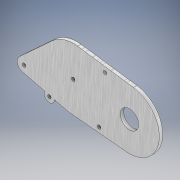
# Autodesk Inventor part: 後脚ギアトレイン5.1
Saved by Autodesk Inventor 2020 (Build 240168000, 168)
## iProperties
Created: 2019-09-03
Part Number: 後脚ギアトレイン5.1
Material: アルミニウム 7075
Document SubType Name: Modeling
Designer: 雪村
Density: 2.81 g/cm^3
Appearance: サテン - ブラシ仕上げ 重厚
Mass: 43.3309 g
Surface Area: 115.743 cm^2
Volume: 15.4203 cm^3
Author: 雪村
Autodesk Inventor part; units mm, degrees
ref_plane "YZ Plane" through (0, 0, 0) normal (1, 0, 0) x (0, 1, 0)
ref_plane "XZ Plane" through (0, 0, 0) normal (0, 1, 0) x (-1, 0, 0)
ref_plane "XY Plane" through (0, 0, 0) normal (0, 0, 1) x (1, 0, 0)
sketch "スケッチ1" plane through (0, 0, 0) normal (0, 0, 1) x (1, 0, 0)
  circle A0 centre (-27.1196, 80) radius 1.5
  circle A1 centre (-27.1196, 80) radius 6
  circle A2 centre (20.6799, 65) radius 1.5
  circle A3 centre (20.6799, 65) radius 6
  circle A4 centre (63.5417, 75.7941) radius 1.5
  circle A5 centre (-68.1796, 83.3936) radius 1.5
  circle A6 centre (-112.5, 70) radius 8.025
  circle A7 centre (112.5, 70) radius 8.025
  arc A8 (109.9686, 44.1235) -> (116.0788, 95.7525) centre (112.5, 70) ccw
  circle A9 centre (-94.9808, 96.6696) radius 4.5
  circle A10 centre (-94.9808, 96.6696) radius 1.5
  circle A11 centre (-83.1426, 57.4965) radius 1.5
  circle A12 centre (-83.1426, 57.4965) radius 4.5
  circle A13 centre (86.1018, 50.9798) radius 4.5
  circle A14 centre (86.1018, 50.9798) radius 1.5
  circle A15 centre (91.2708, 94.6568) radius 1.5
  circle A16 centre (91.2708, 94.6568) radius 4.5
  line L0 (-103.9107, 45.4598) -> (-60.251, 60.7411)
  line L1 (-118.9391, 95.19) -> (-74.1234, 106.646)
  line L2 (-55.9515, 104.0449) -> (-24.0626, 85.1628)
  line L3 (-24.9517, 74.4053) -> (-59.508, 61.015)
  line L4 (116.0788, 95.7525) -> (67.2581, 102.5371)
  line L5 (45.3001, 95.7) -> (16.6263, 69.4235)
  line L6 (19.2049, 59.1841) -> (56.904, 49.6227)
  line L7 (60.9129, 48.9224) -> (109.9686, 44.1235)
  arc A17 (-118.9391, 95.19) -> (-103.9107, 45.4598) centre (-112.5, 70) ccw
  arc A18 (-60.251, 60.7411) -> (-59.508, 61.015) centre (-68.1796, 83.3936) ccw
  arc A19 (-55.9515, 104.0449) -> (-74.1234, 106.646) centre (-68.1796, 83.3936) ccw
  arc A20 (56.904, 49.6227) -> (60.9129, 48.9224) centre (63.5417, 75.7941) ccw
  arc A21 (67.2581, 102.5371) -> (45.3001, 95.7) centre (63.5417, 75.7941) ccw
  point P0 (0, 0)
  point P1 (0, 0)
  point P2 (0, 0)
  dimension "d0" = 3
  dimension "d1" = 12
  dimension "d2" = 3
  dimension "d3" = 12
  dimension "d4" = 3
  dimension "d5" = 3
  dimension "d6" = 16.05
  dimension "d7" = 16.05
  dimension "d8" = 52
  dimension "d9" = 9
  dimension "d10" = 3
  dimension "d11" = 3
  dimension "d12" = 9
  dimension "d13" = 9
  dimension "d14" = 3
  dimension "d15" = 3
  dimension "d16" = 9
  dimension "d17" = 2.0367
  dimension "d18" = 2.0367
  dimension "d19" = 24
  dimension "d20" = 24
  dimension "d21" = 26
  dimension "d22" = 27
  dimension "d23" = 27
  dimension "d24" = 31.9091
  dimension "d25" = 31.9091
  dimension "d26" = 32.5367
  dimension "d27" = 32.5367
  constraints: 22 centre point, 20 tangent, 16 coincident, 16 end point, 16 point on circle, 6 other
  measures "d0" diameter of A0
  measures "d1" diameter of A1
  measures "d2" diameter of A2
  measures "d3" diameter of A3
  measures "d4" diameter of A4
  measures "d5" diameter of A5
  measures "d6" diameter of A6
  measures "d7" diameter of A7
  measures "d8" diameter of A8
  measures "d9" diameter of A9
  measures "d10" diameter of A10
  measures "d11" diameter of A11
  measures "d12" diameter of A12
  measures "d13" diameter of A13
  measures "d14" diameter of A14
  measures "d15" diameter of A15
  measures "d16" diameter of A16
  measures "d19" radius of A19
  measures "d20" radius of A18
  measures "d21" radius of A17
  measures "d22" radius of A20
  measures "d23" radius of A21
  measures "d24" distance of point (-112.5, 70) A9.centre
  measures "d25" distance of A11.centre point (-112.5, 70)
  measures "d26" distance of point (112.5, 70) A15.centre
  measures "d27" distance of A13.centre point (112.5, 70)
extrude "押し出し1" add sketch "スケッチ1" along normal blind 3 contours A3 | A13 | A16 | A3 L5 A21 L4 A8 L7 A20 L6
sketch "スケッチ2" plane through (0, 0, 3) normal (0, 0, 1) x (1, 0, 0)
  arc A0 (56.904, 49.6227) -> (60.9129, 48.9224) centre (63.5417, 75.7941) ccw projected
  line L0 (60.9129, 48.9224) -> (109.9686, 44.1235) projected
  arc A1 (109.9686, 44.1235) -> (116.0788, 95.7525) centre (112.5, 70) ccw projected
  line L1 (116.0788, 95.7525) -> (67.2581, 102.5371) projected
  arc A2 (67.2581, 102.5371) -> (45.3001, 95.7) centre (63.5417, 75.7941) ccw projected
  line L2 (45.3001, 95.7) -> (16.6263, 69.4235) projected
  arc A3 (16.6263, 69.4235) -> (19.2049, 59.1841) centre (20.6799, 65) ccw projected
  line L3 (19.2049, 59.1841) -> (56.904, 49.6227) projected
  circle A4 centre (91.2708, 94.6568) radius 1.5 projected
  circle A5 centre (86.1018, 50.9798) radius 1.5 projected
  circle A6 centre (112.5, 70) radius 8.025 projected
  circle A7 centre (63.5417, 75.7941) radius 1.5 projected
  circle A8 centre (20.6799, 65) radius 1.5 projected
  circle A9 centre (63.5417, 75.7941) radius 27
  circle A10 centre (20.6799, 65) radius 21
  circle A11 centre (34.0051, 86.7414) radius 4.5
  circle A12 centre (34.0051, 86.7414) radius 1.5
  circle A13 centre (42.7132, 52.1631) radius 1.5
  circle A14 centre (42.7132, 52.1631) radius 4.5
  point P0 (0, 0)
  point P1 (38.7185, 54.235)
  point P2 (47.2124, 52.0807)
  point P3 (44.0259, 52.8889)
  point P4 (41.9051, 53.4268)
  point P5 (35.505, 86.7239)
  point P6 (37.9287, 88.9449)
  point P7 (31.4683, 83.0247)
  point P8 (33.892, 85.2457)
  dimension "d30" = 54
  dimension "d31" = 42
  dimension "d32" = 9
  dimension "d33" = 3
  dimension "d34" = 3
  dimension "d35" = 9
  constraints: 6 centre point, 4 coincident, 4 tangent
  measures "d30" diameter of A9
  measures "d31" diameter of A10
  measures "d32" diameter of A11
  measures "d33" diameter of A12
  measures "d34" diameter of A13
  measures "d35" diameter of A14
extrude "押し出し2" add sketch "スケッチ2" against normal blind 3 contours A14 L3 A13
sketch "スケッチ3" plane through (0, 0, 3) normal (0, 0, 1) x (1, 0, 0)
  line L0 (47.2124, 52.0807) -> (56.904, 49.6227) projected
  arc A0 (56.904, 49.6227) -> (60.9129, 48.9224) centre (63.5417, 75.7941) ccw projected
  line L1 (60.9129, 48.9224) -> (109.9686, 44.1235) projected
  arc A1 (109.9686, 44.1235) -> (116.0788, 95.7525) centre (112.5, 70) ccw projected
  line L2 (116.0788, 95.7525) -> (67.2581, 102.5371) projected
  arc A2 (67.2581, 102.5371) -> (45.3001, 95.7) centre (63.5417, 75.7941) ccw projected
  line L3 (45.3001, 95.7) -> (16.6263, 69.4235) projected
  arc A3 (16.6263, 69.4235) -> (19.2049, 59.1841) centre (20.6799, 65) ccw projected
  circle A4 centre (91.2708, 94.6568) radius 1.5 projected
  circle A5 centre (86.1018, 50.9798) radius 1.5 projected
  circle A6 centre (112.5, 70) radius 8.025 projected
  circle A7 centre (63.5417, 75.7941) radius 1.5 projected
  circle A8 centre (20.6799, 65) radius 1.5 projected
  circle A9 centre (34.0051, 86.7414) radius 1.5
  circle A10 centre (42.7132, 52.1631) radius 1.5
  arc A11 (38.7185, 54.235) -> (47.2124, 52.0807) centre (42.7132, 52.1631) ccw projected
  line L4 (19.2049, 59.1841) -> (38.7185, 54.235) projected
  point P0 (0, 0)
  point P1 (41.9051, 53.4268)
  point P2 (44.0259, 52.8889)
  point P3 (35.505, 86.7239)
  point P4 (33.892, 85.2457)
  dimension "d38" = 3
  dimension "d39" = 3
  constraints: 2 centre point
  measures "d38" diameter of A9
  measures "d39" diameter of A10
extrude "押し出し3" cut sketch "スケッチ3" against normal blind 3 contours A9 L3 | A10 picked at (33.6626, 86.26)
sketch "スケッチ4" plane through (0, 0, 0) normal (0, 0, -1) x (-1, 0, 0)
  circle A0 centre (-63.5417, 75.7941) radius 1.5 projected
  circle A1 centre (-20.6799, 65) radius 1.5 projected
  circle A2 centre (-20.6799, 65) radius 6
  circle A3 centre (-20.6799, 65) radius 4
  circle A4 centre (-63.5417, 75.7941) radius 4
  circle A5 centre (-63.5417, 75.7941) radius 6
  point P0 (0, 0)
  dimension "d42" = 12
  dimension "d43" = 8
  dimension "d44" = 8
  dimension "d45" = 12
  constraints: 4 centre point, 4 coincident
  measures "d42" diameter of A2
  measures "d43" diameter of A3
  measures "d44" diameter of A4
  measures "d45" diameter of A5
extrude "押し出し4" cut sketch "スケッチ4" against normal blind 0.5 contours A2 | A5
fillet "フィレット1" radius 1 2 edges at (19.2049, 59.1841, 0.25) (16.6263, 69.4235, 0.25)
